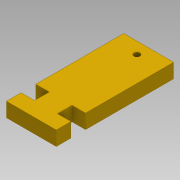
# Autodesk Inventor part: В. шарн. - держатель смартфона
Saved by Autodesk Inventor 2018 (Build 220112000, 112)
## iProperties
Created: 2020-02-22
Part Number: В. шарн. - держатель смартфона
Material: Типовые
Document SubType Name: Modeling
Designer: Leancher
Density: 1 g/cm^3
Appearance: По умолчанию
Author: Leancher
Autodesk Inventor part; units mm, degrees
ref_plane "YZ Plane" through (0, 0, 0) normal (1, 0, 0) x (0, 1, 0)
ref_plane "XZ Plane" through (0, 0, 0) normal (0, 1, 0) x (-1, 0, 0)
ref_plane "XY Plane" through (0, 0, 0) normal (0, 0, 1) x (1, 0, 0)
sketch "Эскиз1" plane through (0, 0, 0) normal (0, 0, 1) x (1, 0, 0)
  line L0 (-5.1487, -13.4444) -> (-9.7487, -13.4444)
  line L1 (-9.7487, -13.4444) -> (-9.7487, -18.4444)
  line L2 (-9.7487, -18.4444) -> (7.2513, -18.4444)
  line L3 (7.2513, -18.4444) -> (7.2513, -13.4444)
  line L4 (7.2513, -13.4444) -> (2.6513, -13.4444)
  line L5 (2.6513, -13.4444) -> (2.6513, -8.4651)
  line L6 (2.6513, -8.4651) -> (7.2513, -8.4651)
  line L7 (7.2513, -8.4651) -> (7.2513, 21.5556)
  line L8 (7.2513, 21.5556) -> (-9.7487, 21.5556)
  line L9 (-9.7487, 21.5556) -> (-9.7487, -8.4237)
  line L10 (-9.7487, -8.4237) -> (-5.1487, -8.4237)
  line L11 (-5.1487, -8.4237) -> (-5.1487, -13.4444)
  circle A0 centre (-1.2487, 17.5556) radius 1
  constraints: 24 end point, 1 centre point
extrude "Выдавливание1" add sketch "Эскиз1" along normal blind 4.9
